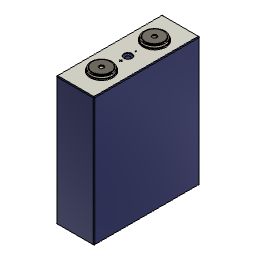
ogniwo (Autodesk Fusion 360 archive; units mm, degrees)
design "ogniwo" references "Śruba z łbem niskim z gniazdem sześciokątnym ASME B18.3.1M — M5x0.8 x 8 Stal klasy 2 Płaszczyzna"
Autodesk Fusion 360 part; units mm, degrees
note: some values were not read from the file. Chosen so that the rebuilt part matches the saved one: which bodies a step acts on; how an offset face is resized. Set by a fixed rule: which sketch regions a step uses.
sketch "Szkic1" plane through (0, 0, 0) normal (0, 0, 1) x (1, 0, 0)
  line L0 (0, 0) -> (50, 0)
  line L1 (50, 0) -> (50, 140)
  line L2 (50, 140) -> (0, 140)
  line L3 (0, 140) -> (0, 0)
  dimension "d1" = 50
  dimension "d2" = 140
  constraint horizontal L0
  constraint vertical L1
  constraint horizontal L2
  constraint vertical L3
  constraint coincident L0.start L3.end
  measures "d1" distance of L0.start L0.end
  measures "d2" distance of L0.start L2.end
extrude "Wyciągnięcie proste1" add sketch "Szkic1" along normal blind 170 makes body 1
ref_plane "Płaszczyzna konstrukcyjna1" through (25, 70, 170) normal (0, 0, 1) x (1, 0, 0)
sketch "Szkic2" plane through (0, 0, 170) normal (0, 0, 1) x (1, 0, 0)
  line L0 (0, 70) -> (50, 70) construction
  line L1 (0, 140) -> (50, 70) construction
  line L2 (0, 0) -> (50, 70) construction
  line L3 (0, 70) -> (50, 140) construction
  line L4 (0, 70) -> (50, 0) construction
  circle A0 centre (25, 105) radius 15
  circle A1 centre (25, 105) radius 14
  circle A2 centre (25, 105) radius 12.5
  dimension "d6" = 30
  dimension "d7" = 28
  dimension "d8" = 25
  constraint horizontal L0
  constraint coincident L2.start origin
  constraint parallel L2 L3
  constraint midpoint L3 A0.centre
  constraint concentric A0 A1
  constraint concentric A0 A2
  measures "d6" diameter of A0
  measures "d7" diameter of A1
  measures "d8" diameter of A2
extrude "Wyciągnięcie proste2" add sketch "Szkic2" along normal blind 5 contours A2 bodies 1
extrude "Wyciągnięcie proste3" add sketch "Szkic2" along normal blind 4 contours A1 bodies 1
extrude "Wyciągnięcie proste4" add sketch "Szkic2" along normal blind 1.5 contours A0 bodies 1
split "Podział1" by plane through (0, 0, 170) normal (0, 0, 1) bodies 1 makes body 2 at (24.0728, 103.3941, 175)
ref_plane "Płaszczyzna konstrukcyjna2" through (25, 70, 85) normal (0, 1, 0) x (-1, 0, 0)
mirror "Odbij1" about plane through (25, 70, 85) normal (0, 1, 0) of bodies 2 makes body 3
chamfer "Fazowanie1" distance 0.5 angle 45 2 edges at (13.3459, 39.5202, 175) (13.3459, 100.4798, 175) on bodies 2 3
sketch "Szkic3" plane through (0, 0, 175) normal (0, 0, 1) x (-1, 0, 0)
  circle A0 centre (-25, -35) radius 12
  circle A1 centre (-25, -35) radius 3
  circle A2 centre (-25, -105) radius 3
  dimension "d18" = 6
  dimension "d19" = 6
  constraint concentric A0 A1
  measures "d18" diameter of A1
  measures "d19" diameter of A2
extrude "Wyciągnięcie proste5" cut sketch "Szkic3" against normal blind 10 contours A1 | A2 bodies 1 2 3
combine "Kombinacja1" operation add target body 1 tool bodies 2 3
thread "Gwint1" "ISO Metric profile 6.0 M6x1 6H" major diameter 6.147 minor diameter 5.035 pitch 1 angle 60 resizes the face on face at (22.0149, 35.2987, 171.6667) on bodies 1
thread "Gwint2" "ISO Metric profile 6.0 M6x1 6H" major diameter 6.147 minor diameter 5.035 pitch 1 angle 60 resizes the face on face at (22.1809, 106.0261, 168.3333) on bodies 1
chamfer "Fazowanie2" distance 0.5 angle 45 2 edges at (27.3471, 34.0896, 175) (27.3471, 104.0896, 175) on bodies 1
fillet "Zaokrąglenie1" radius 0.15 4 edges at (11.9474, 40.0626, 174) (11.0151, 40.4242, 171.5) (11.9474, 99.9374, 174) (11.0151, 99.5758, 171.5) on bodies 1
fillet "Zaokrąglenie2" radius 1 5 faces at (50, 46.6667, 56.6667) (33.3333, 140, 113.3333) (0, 93.3333, 56.6667) (16.6667, 0, 113.3333) (16.6667, 93.3333, 0) on bodies 1
sketch "Szkic4" plane through (0, 0, 170) normal (0, 0, 1) x (-1, 0, 0)
  line L0 (-49, -1) -> (-49, -139)
  line L1 (-49, -139) -> (-1, -139)
  line L2 (-1, -139) -> (-1, -1)
  line L3 (-1, -1) -> (-49, -1)
  line L4 (-20.0882, -84.9291) -> (-20.0683, -55.0033) construction
  line L5 (-20.0683, -55.0033) -> (-29.9317, -54.9967) construction
  line L6 (-29.9317, -54.9967) -> (-29.9516, -84.9225) construction
  line L7 (-29.9516, -84.9225) -> (-20.0882, -84.9291) construction
  circle A0 centre (-25, -105) radius 15
  circle A1 centre (-25, -35) radius 15
  dimension "d31" = 5
  text T0 "-         +" font "Arial" height 5 align centre middle in box 29.9258 x 9.8634 at (-20.0882, -84.9291) x (0.000664, 1) y (-1, 0.000664) spacing 1
extrude "Wyciągnięcie proste6" cut sketch "Szkic4" against normal blind 0.5 text T0 bodies 1
sketch "Szkic5" plane through (0, 0, 170) normal (0, 0, 1) x (-1, 0, 0)
  line L0 (-25.1259, -59.6934) -> (-23.7548, -59.6943)
  line L1 (-23.7548, -59.6943) -> (-23.7552, -60.2741)
  line L2 (-23.7552, -60.2741) -> (-25.1263, -60.2732)
  line L3 (-25.1263, -60.2732) -> (-25.1272, -61.634)
  line L4 (-25.1272, -61.634) -> (-25.7002, -61.6337)
  line L5 (-25.7002, -61.6337) -> (-25.6993, -60.2728)
  line L6 (-25.6993, -60.2728) -> (-27.0601, -60.2719)
  line L7 (-27.0601, -60.2719) -> (-27.0597, -59.6921)
  line L8 (-27.0597, -59.6921) -> (-25.6989, -59.693)
  line L9 (-25.6989, -59.693) -> (-25.698, -58.3322)
  line L10 (-25.698, -58.3322) -> (-25.125, -58.3325)
  line L11 (-25.125, -58.3325) -> (-25.1259, -59.6934)
  line L12 (-25.0778, -79.7071) -> (-24.4605, -79.7075)
  line L13 (-24.4605, -79.7075) -> (-24.4617, -81.5936)
  line L14 (-24.4617, -81.5936) -> (-25.079, -81.5932)
  line L15 (-25.079, -81.5932) -> (-25.0778, -79.7071)
  line L16 (-49, -1) -> (-49, -139)
  line L17 (-49, -139) -> (-1, -139)
  line L18 (-1, -139) -> (-1, -1)
  line L19 (-1, -1) -> (-49, -1)
  circle A0 centre (-25, -70) radius 5
  circle A1 centre (-25, -105) radius 15
  circle A2 centre (-25, -35) radius 15
  dimension "d34" = 10
  measures "d34" diameter of A0
extrude "Wyciągnięcie proste7" cut sketch "Szkic5" against normal blind 2 contours A0 bodies 1
fillet "Zaokrąglenie3" radius 2 1 edges at (29.6616, 68.1919, 168) on bodies 1
fillet "Zaokrąglenie4" radius 0.5 1 edges at (29.6616, 68.1919, 170) on bodies 1
split "Podział2" by plane through (0, 140, 174) normal (0, 0, 1) bodies 1 makes body 4 at (33.9499, 34.2539, 175) makes body 5 at (21.1712, 96.8761, 175)
split "Podział3" by plane through (0, 0, 170) normal (0, 0, 1) bodies 1 makes body 6 at (21.0878, 96.7318, 174) makes body 7 at (34.126, 35.621, 174)
other "Śruba1"
other "Śruba2"
component "ogniwo v6" placed x (1, 0, 0) y (0, 1, 0) z (0, 0, 1) at (0, 0, 0)
component "ogniwo v6" placed x (1, 0, 0) y (0, 1, 0) z (0, 0, 1) at (0, 0, 0)
component "ogniwo" placed x (1, 0, 0) y (0, 1, 0) z (0, 0, 1) at (0, 0, 0)

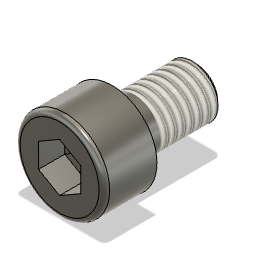
design "Śruba z łbem niskim z gniazdem sześciokątnym ASME B18.3.1M — M5x0.8 x 8 Stal klasy 2 Płaszczyzna"
description: Śruba z łbem niskim z gniazdem sześciokątnym ASME B18.3.1M — M5x0.8 x 8
Autodesk Fusion 360 part; units mm, degrees
sketch "Sketch1" plane through (0, 0, 0) normal (0, 1, 0) x (1, 0, 0)
  line L0 (-2.5, 0) -> (-2.5, 8)
  line L1 (-2.5, 8) -> (0, 8)
  line L2 (0, 8) -> (0, -5)
  line L3 (-2.5, 0) -> (-4.25, 0)
  line L4 (-4.25, 0) -> (-4.25, -5)
  line L5 (-4.25, -5) -> (0, -5)
  dimension "d9" = 5
  dimension "d66" = 8.5
  dimension "d68" = 8
  dimension "d79" = 5
  constraint perpendicular L0 L1
  constraint collinear origin L1.end L2.end
  constraint perpendicular L0 L3
  constraint coincident origin L3
  constraint vertical L0
  constraint vertical L2
  constraint parallel L2 L4
  constraint coincident L2 L5.end
  constraint perpendicular L2 L5
  measures "d68" distance of origin L1.end
  measures "d79" distance of L3.end L4.end
revolve "Revolve1" add sketch "Sketch1" angle 360 about axis through (0, 0, -8) along (0, 0, 1)
ref_plane "WorkPlane1" through (0, 0, 5) normal (0, 0, 1) x (1, 0, 0)
sketch "Sketch6" plane through (0, 0, 5) normal (0, 0, 1) x (1, 0, 0)
  line L0 (-2, 0) -> (2, 0) construction
  line L1 (0, 0) -> (-2, 1.1547)
  line L2 (-2, -1.1547) -> (-2, 1.1547)
  line L3 (-2, -1.1547) -> (0, 0)
  dimension "d72" = 4
  dimension "d100" = 150
  constraint horizontal L0
  constraint midpoint L1.start L0
  constraint coincident L1.start L3.end
  constraint perpendicular L0 L2
  constraint midpoint L0.start L2
  constraint coincident L1.end L2.end
  measures "d72" distance of L0.start L0.end
  measures "d100" angle of L0 L1
extrude "Extrude1" cut sketch "Sketch6" against normal blind 2.5
pattern_circular "C-Pattern1" count 6 over 360 about axis through (0, 0, 1.75) along (0, 0, 1) of "Extrude1"
extrude "Extrude2" cut 1 faces at (-0.6667, 0.3849, 2.5) along direction (0, 0, -1) blind 2.5 draft -85
thread "Thread2" "ANSI Metric M Profile 5.0 M5x0.8 4g6g" major diameter 4.901 minor diameter 4.007 pitch 0.8 angle 60 resizes the face on face at (-2.4969, 0.1246, -2.6667)
fillet "Fillet4" radius 0.5 1 edges at (-3.9624, 1.5369, 5)
sketch "Sketch7" plane through (0, 0, 0) normal (0, 1, 0) x (1, 0, 0)
  line L0 (-2.55, 8) -> (-2.55, 7.5092)
  line L1 (-2.55, 7.5092) -> (-2.0092, 8)
  line L2 (0, 8) -> (0, -5)
  line L3 (-2.55, 8) -> (0, 8)
  dimension "d92" = 0.4908
  dimension "d98" = 2.0092
  dimension "d99" = 2.55
  constraint coincident L2.start L3.end
  constraint perpendicular L2 L3
  constraint coincident L1.end L3
  constraint perpendicular L0 L3
  measures "d92" vertical distance of L0.end L1.end
  measures "d98" horizontal distance of origin L1.end
  measures "d99" distance of origin L0
revolve "Revolve3" cut sketch "Sketch7" angle 360 about axis through (0, 0, 1.75) along (0, 0, 1)
equation "d9 = adsk_nomdia"
equation "adsk_nomlen = 8.00 mm"
equation "adsk_headh = 5.00 mm"
equation "adsk_headdia = 8.50 mm"
equation "adsk_nomdia = 5.00 mm"
equation "adsk_philwidth = 4.00 mm"
equation "d31 = -adsk_phildepth"
equation "adsk_phildepth = 2.50 mm"
equation "d66 = adsk_headdia"
equation "d68 = adsk_nomlen"
equation "d71 = adsk_headh"
equation "d72 = adsk_philwidth"
equation "d76 = -adsk_phildepth"
equation "d79 = adsk_headh"
equation "adsk_thrlen = 5.90924 mm"
equation "d84 = adsk_thrlen"
equation "d86 = adsk_nomdia * 0.1"
equation "d92 = adsk_startlen"
equation "adsk_startlen = 0.49076 mm"
equation "adsk_endpointdia = 4.01848 mm"
equation "d98 = adsk_endpointdia / 2"
equation "d99 = adsk_nomdia * 0.51"
